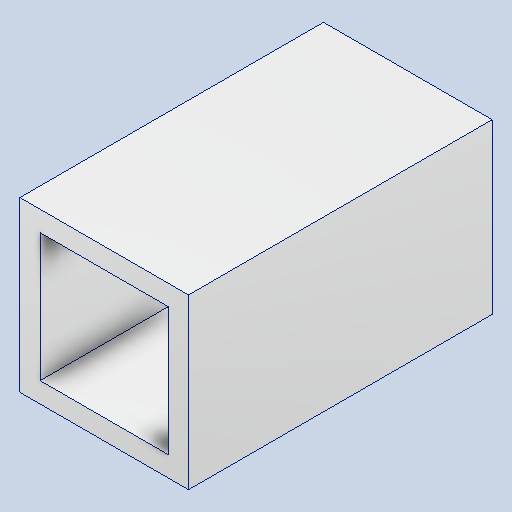
# Autodesk Inventor part: P601
Saved by Autodesk Inventor 2023 (Build 270158000, 158)
## iProperties
Created: 2022-08-22
Part Number: P601
Material: Aluminum 6061
Document SubType Name: Modeling
Designer: D.C. Eksteen
Density: 2.7 g/cm^3
Appearance: Aluminum - Flat
Mass: 19.2846 g
Surface Area: 75.8565 cm^2
Volume: 7.14244 cm^3
Author: D.C. Eksteen
Title: REAR FRONT PLAIN RISER
Autodesk Inventor part; units mm, degrees
ref_plane "YZ Plane" through (0, 0, 0) normal (1, 0, 0) x (0, 1, 0)
ref_plane "XZ Plane" through (0, 0, 0) normal (0, 1, 0) x (-1, 0, 0)
ref_plane "XY Plane" through (0, 0, 0) normal (0, 0, 1) x (1, 0, 0)
sketch "Sketch1" plane through (0, 0, 0) normal (0, 0, 1) x (1, 0, 0)
  line L0 (0, 0) -> (25, 0)
  line L1 (25, 0) -> (25, 25)
  line L2 (25, 25) -> (0, 25)
  line L3 (0, 25) -> (0, 0)
  line L4 (3, 22) -> (22, 22)
  line L5 (22, 22) -> (22, 3)
  line L6 (22, 3) -> (3, 3)
  line L7 (3, 3) -> (3, 22)
  dimension "d0" = 25
  dimension "d1" = 25
  dimension "d2" = 3
  constraints: 16 end point, 4 parallel, 2 perpendicular, 1 horizontal, 3 other
  measures "d0" distance of L2.end L1.end
  measures "d1" distance of L1.end L0.end
  measures "d2" distance between parallel lines of L2 L4
extrude "Extrusion1" add sketch "Sketch1" against normal blind 300
sketch "Sketch2" plane through (25, 0, 0) normal (1, 0, 0) x (0, 0, -1)
  line L0 (0, 0) -> (0, 25) projected
  line L1 (0, 0) -> (300, 0) projected
  line L2 (300, 25) -> (300, 0) projected
  line L3 (0, 25) -> (300, 25) projected
  line L4 (0, 25) -> (300, 25) projected
  line L5 (48.3423, 25) -> (60, 0)
  line L6 (0, 0) -> (300, 0) projected
  line L7 (0, 0) -> (-11.6577, 25)
  line L8 (-11.6577, 25) -> (48.3423, 25)
  line L9 (255, 0) -> (230, 25)
  line L10 (255, 0) -> (300, 0)
  line L11 (0, 3) -> (300, 3) projected
  line L12 (275, 25) -> (230, 25)
  line L13 (255, 0) -> (255, 25)
  line L14 (242.5, 12.5) -> (255, 25)
  line L15 (255, 0) -> (255, 3)
  line L16 (0, 3) -> (300, 3) projected
  line L17 (252, 3) -> (255, 3)
  line L18 (252, 3) -> (255, 0)
  point P0 (58.6011, 3)
  point P1 (255, 3)
  point P2 (255, 3)
  dimension "d6" = 65
  dimension "d10" = 60
  dimension "d11" = 45
  dimension "d21" = 70
  constraints: 22 end point, 10 point on line, 3 collinear, 2 parallel, 1 horizontal, 1 midpoint, 1 perpendicular
  measures "d6" angle of L1 L5
  measures "d10" distance of L5.end L6.start
  measures "d11" angle of L1 L9
  measures "d21" distance from line of L2 L9.end
extrude "Extrusion2" cut sketch "Sketch2" against normal blind 300 contours L13 L11 L2 L1 | L13 L3 L2 L11 keep common part
body "Solid1"
